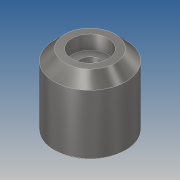
# Autodesk Inventor part: 200-60-DIFFERENTIAL-CONNECTOR-03
Saved by Autodesk Inventor 2018.2 (Build 222227000, 227)
## iProperties
Manager: feesmrt
Company: FRANC0R
Created: 2017-12-05
Part Number: 200-60-DIFFERENTIAL-CONNECTOR-03
Material: Edelstahl
Document SubType Name: Modeling
Designer: feesmrt
Density: 8 g/cm^3
Appearance: Halbpoliert
Project: Rescue Robot
Cost Center: -
Engineer: feesmrt
Authority: feesmrt
Description: Differential Connector Cap
Stock Number: 200-60-DIFFERENTIAL-CONNECTOR-03
Author: feesmrt
Subject: Rescue Robot
Title: Differential Connector Cap
Revision Number: 1
Autodesk Inventor part; units mm, degrees
ref_plane "YZ Plane" through (0, 0, 0) normal (1, 0, 0) x (0, 1, 0)
ref_plane "XZ Plane" through (0, 0, 0) normal (0, 1, 0) x (-1, 0, 0)
ref_plane "XY Plane" through (0, 0, 0) normal (0, 0, 1) x (1, 0, 0)
sketch "Skizze2" plane through (0, 0, 0) normal (0, 0, 1) x (1, 0, 0)
  line L0 (0, 14) -> (0, -14) construction
  line L1 (-14, 0) -> (14, 0) construction
  circle A0 centre (0, 0) radius 10
  dimension "d0" = 20
  constraints: 1 centre point, 1 coincident
  measures "d0" diameter of A0
extrude "Grundkörper" add sketch "Skizze2" along normal blind 20
sketch "Skizze3" plane through (0, 0, 0) normal (0, 0, -1) x (-1, 0, 0)
  line L0 (0, -14) -> (0, 14) projected
  line L1 (-14, 0) -> (14, 0) projected
  point P0 (0, 0)
  point P1 (0, 0)
  constraints: 1 coincident
hole "12H7_Passbohrung" at (0, 0, 0) direction (0, 0, 1) diameter 12 depth 10
sketch "Skizze4" plane through (0, 0, 20) normal (0, 0, 1) x (1, 0, 0)
  line L0 (0, 14) -> (0, -14) construction
  line L1 (-14, 0) -> (14, 0) construction
  point P0 (0, 0)
  point P1 (0, 0)
  constraints: 1 coincident
hole "DIN7984_M5_Bohrung" at (0, 0, 20) direction (0, 0, -1) diameter 5.5 end through all counterbore diameter 10 counterbore depth 3.9
chamfer "Fase_Deckel" distance 3 angle 45 1 edges at (-10, 0, 20)
chamfer "Fase_Allgemein" distance 0.5 angle 45 2 edges at (0, -6, 0) (-10, 0, 0)
